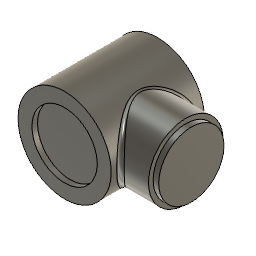
link5 (Autodesk Fusion 360 design; units mm, degrees)
part number: 2025-12-14-18-36-43-908
Autodesk Fusion 360 part; units mm, degrees
sketch "Sketch1" plane through (0, 0, 0) normal (0, 1, 0) x (1, 0, 0)
  circle A0 centre (0, 0) radius 25
  dimension "d1" = 50
  constraint coincident A0.centre origin
  measures "d1" diameter of A0
extrude "Extrude2" add sketch "Sketch1" along normal mid plane 50
sketch "Sketch2" plane through (0, -25, 0) normal (0, -1, 0) x (1, 0, 0)
  circle A0 centre (0, 0) radius 25
  circle A1 centre (0, 0) radius 17.5
  dimension "d6" = 35
  constraint coincident A0.centre A1.centre
  measures "d6" diameter of A1
extrude "Extrude3" cut sketch "Sketch2" against normal blind 3 contours A1
mirror "Mirror1" about plane through (0, 0, 0) normal (0, 1, 0) of "Extrude3"
sketch "Sketch3" plane through (0, 0, 0) normal (1, 0, 0) x (0, 1, 0)
  circle A0 centre (0, 0) radius 20
  dimension "d11" = 40
  constraint coincident A0.centre origin
  measures "d11" diameter of A0
extrude "Extrude4" add sketch "Sketch3" along normal blind 40
sketch "Sketch4" plane through (40, 0, 0) normal (1, 0, 0) x (0, 1, 0)
  circle A0 centre (0, 0) radius 20
  circle A1 centre (0, 0) radius 17.5
  dimension "d14" = 35
  constraint coincident A0.centre A1.centre
  measures "d14" diameter of A1
extrude "Extrude5" add sketch "Sketch4" along normal blind 3 contours A1
fillet "Fillet1" radius 2 1 edges at (15, 0, 20)
